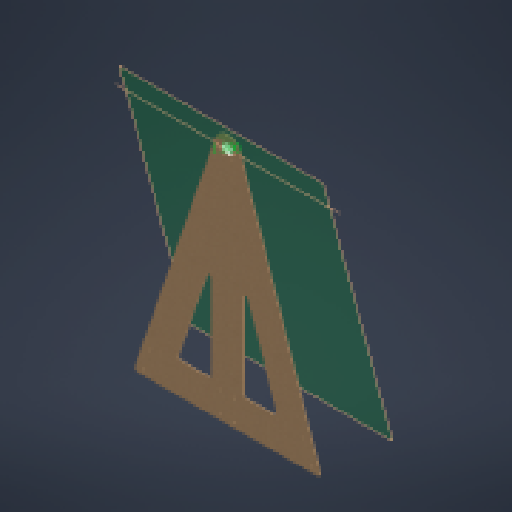
# Autodesk Inventor part: FrameTop
Saved by Autodesk Inventor 2024.1 (Build 281209000, 209)
## iProperties
Created: 2023-10-16
Part Number: FrameTop
Material: MDF Medium Density Fiberboard
Document SubType Name: Modeling
Designer: Brandon
Density: 0.8 g/cm^3
Appearance: Cardboard - Corrugated
Author: Brandon
Autodesk Inventor part; units mm, degrees
ref_plane "YZ Plane" through (0, 0, 0) normal (1, 0, 0) x (0, 1, 0)
ref_plane "XZ Plane" through (0, 0, 0) normal (0, 1, 0) x (-1, 0, 0)
ref_plane "XY Plane" through (0, 0, 0) normal (0, 0, 1) x (1, 0, 0)
sketch "Sketch1" plane through (0, 0, 0) normal (0, 0, 1) x (1, 0, 0)
  circle A0 centre (-11, 0) radius 11 projected
  circle A1 centre (-11, 0) radius 31.75
  line L0 (217.6, 31.75) -> (-239.6, 31.75)
  line L1 (-239.6, 31.75) -> (-239.6, -577.85)
  line L2 (-239.6, -577.85) -> (217.6, -577.85)
  line L3 (217.6, -577.85) -> (217.6, 31.75)
  line L4 (217.6, -577.85) -> (19.0819, 10.156)
  line L5 (-239.6, -577.85) -> (-41.0819, 10.156)
  line L6 (27.1, -501.65) -> (111.4484, -501.65)
  line L7 (111.4484, -501.65) -> (27.1, -251.8121)
  line L8 (27.1, -251.8121) -> (27.1, -501.65)
  line L9 (-11, 0) -> (-11, -6.454)
  line L10 (-49.1, -501.65) -> (-133.4484, -501.65)
  line L11 (-133.4484, -501.65) -> (-49.1, -251.8121)
  line L12 (-49.1, -251.8121) -> (-49.1, -501.65)
  circle A2 centre (193.2059, -565.15) radius 2
  circle A3 centre (176.0552, -514.35) radius 2
  circle A4 centre (8.05, -514.35) radius 2
  circle A5 centre (8.05, -565.15) radius 2
  circle A6 centre (-215.2059, -565.15) radius 2
  circle A7 centre (-198.0552, -514.35) radius 2
  circle A8 centre (-30.05, -514.35) radius 2
  circle A9 centre (-30.05, -565.15) radius 2
  circle A10 centre (-28.78, 0) radius 2
  circle A11 centre (-19.89, -15.3979) radius 2
  circle A12 centre (-2.11, -15.3979) radius 2
  circle A13 centre (6.78, 0) radius 2
  circle A14 centre (-2.11, 15.3979) radius 2
  circle A15 centre (-19.89, 15.3979) radius 2
  point P0 (0, 0)
  point P1 (-11, 31.75)
  point P2 (-11, -3.227)
  dimension "d0" = 63.5
  dimension "d1" = 457.2
  dimension "d2" = 609.6
  dimension "d3" = 76.2
  dimension "d4" = 76.2
  dimension "d5" = 38.1
  dimension "d6" = 4
  dimension "d7" = 4
  dimension "d8" = 4
  dimension "d9" = 4
  dimension "d10" = 12.7
  dimension "d11" = 12.7
  dimension "d12" = 19.05
  dimension "d13" = 19.05
  dimension "d14" = 19.05
  dimension "d15" = 4
  dimension "d16" = 17.78
  dimension "d19" = 360
  constraints: 26 end point, 15 centre point, 7 symmetric about line, 4 horizontal alignment, 3 parallel, 3 tangent, 2 horizontal, 2 midpoint, 2 perpendicular, 2 point on circle, 2 vertical alignment, 1 coincident, 1 vertical, 17 other
  measures "d0" diameter of A1
  measures "d1" distance of L2.end L1.end
  measures "d2" distance of L1.end L0.end
  measures "d3" distance between parallel lines of L4 L7
  measures "d4" distance between parallel lines of L2 L6
  measures "d5" distance from line of point (-11, 0) L8
  measures "d6" diameter of A2
  measures "d7" diameter of A3
  measures "d8" diameter of A4
  measures "d9" diameter of A5
  measures "d10" distance from line of L6 A4.centre
  measures "d11" distance from line of L2 A5.centre
  measures "d12" horizontal distance of A4.centre point (-11, -3.227)
  measures "d13" distance from line of L4 A3.centre
  measures "d14" distance from line of L4 A2.centre
  measures "d15" diameter of A10
  measures "d16" distance of point (-11, 0) A10.centre
extrude "Extrusion1" add sketch "Sketch1" against normal blind 3.175 contours A1 | A1 L4 L2 L5
fillet "Fillet1" radius 6.35 8 edges at (27.1, -251.8121, -1.5875) (-49.1, -251.8121, -1.5875) (111.4484, -501.65, -1.5875) (217.6, -577.85, -1.5875) (27.1, -501.65, -1.5875) (-49.1, -501.65, -1.5875) (-133.4484, -501.65, -1.5875) (-239.6, -577.85, -1.5875)
ref_plane "Work Plane1" through (-28.78, 0, -3.175) normal (0, 0.2588, -0.9659) x (1, 0, 0)
sketch "Sketch2" plane through (-28.78, 0, -3.175) normal (0, 0.2588, -0.9659) x (1, 0, 0)
  ellipse E0 centre (17.78, 0) end of major axis (6.7038, 0) minor radius 10.6988
  circle A0 centre (17.78, 0) radius 12.7
  dimension "d26" = 25.4
  constraints: 1 centre point, 1 coincident, 3 other
  measures "d26" diameter of A0
sketch "Sketch3" plane through (0, 0, -3.175) normal (0, 0, -1) x (-1, 0, 0)
  ellipse E0 centre (11, 0) end of major axis (-1.7, 0) minor radius 12.2673 projected
  point P0 (0, 0)
  constraints: 1 other
extrude "Extrusion2" cut sketch "Sketch3" against normal through all
body "Solid1"
